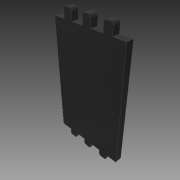
# Autodesk Inventor part: spool_stand_brace_middle_b
Saved by Autodesk Inventor 2014 (Build 180170000, 170)
## iProperties
Created: 2014-04-08
Part Number: spool_stand_brace_middle_b
Material: Plywood, Finish
Document SubType Name: Modeling
Designer: buben
Density: 0.552 g/cm^3
Appearance: Anodized - Dark Gray
Author: buben
Autodesk Inventor part; units mm, degrees
ref_plane "YZ Plane" through (0, 0, 0) normal (1, 0, 0) x (0, 1, 0)
ref_plane "XZ Plane" through (0, 0, 0) normal (0, 1, 0) x (-1, 0, 0)
ref_plane "XY Plane" through (0, 0, 0) normal (0, 0, 1) x (1, 0, 0)
sketch "Sketch1" plane through (0, 0, 0) normal (0, 1, 0) x (-1, 0, 0)
  line L0 (0, 0) -> (-68.411, 0)
  line L1 (-68.411, 0) -> (-68.411, -110)
  line L2 (-68.411, -110) -> (0, -110)
  line L3 (0, -110) -> (0, 0)
  dimension "d0" = 110
  dimension "d1" = 68.411
  constraints: 8 end point, 2 parallel, 1 horizontal, 1 perpendicular
  measures "d0" distance of L2.end L0.start
  measures "d1" distance of L0.start L0.end
extrude "Extrusion1" add sketch "Sketch1" along normal blind 6.5
sketch "Sketch2" plane through (0, 6.5, 0) normal (0, 1, 0) x (1, 0, 0)
  line L0 (68.411, 0) -> (68.411, 110) projected
  line L1 (68.411, 110) -> (0, 110) projected
  line L2 (0, 110) -> (0, 0) projected
  line L3 (11.1027, 110) -> (19.1027, 110)
  line L4 (19.1027, 110) -> (19.1027, 114.5)
  line L5 (17.1027, 116.5) -> (13.1027, 116.5)
  line L6 (11.1027, 114.5) -> (11.1027, 110)
  line L7 (30.2055, 110) -> (38.2055, 110)
  line L8 (38.2055, 110) -> (38.2055, 114.5)
  line L9 (36.2055, 116.5) -> (32.2055, 116.5)
  line L10 (30.2055, 114.5) -> (30.2055, 110)
  line L11 (49.3082, 110) -> (57.3082, 110)
  line L12 (57.3082, 110) -> (57.3082, 114.5)
  line L13 (55.3082, 116.5) -> (51.3082, 116.5)
  line L14 (49.3082, 114.5) -> (49.3082, 110)
  arc A0 (13.1027, 116.5) -> (11.1027, 114.5) centre (13.1027, 114.5) ccw
  arc A1 (19.1027, 114.5) -> (17.1027, 116.5) centre (17.1027, 114.5) ccw
  arc A2 (32.2055, 116.5) -> (30.2055, 114.5) centre (32.2055, 114.5) ccw
  arc A3 (38.2055, 114.5) -> (36.2055, 116.5) centre (36.2055, 114.5) ccw
  arc A4 (51.3082, 116.5) -> (49.3082, 114.5) centre (51.3082, 114.5) ccw
  arc A5 (57.3082, 114.5) -> (55.3082, 116.5) centre (55.3082, 114.5) ccw
  line L15 (11.1027, 112.25) -> (0, 112.25) construction
  line L16 (19.1027, 112.25) -> (30.2055, 112.25) construction
  line L17 (38.2055, 112.25) -> (49.3082, 112.25) construction
  line L18 (57.3082, 112.25) -> (68.411, 112.25) construction
  line L19 (0, 55) -> (68.411, 55) construction
  line L20 (0, 0) -> (68.411, 0) projected
  line L21 (68.411, 0) -> (68.411, 110) projected
  line L22 (68.411, 110) -> (0, 110) projected
  line L23 (0, 110) -> (0, 0) projected
  line L24 (11.1027, 0) -> (19.1027, 0)
  line L25 (19.1027, 0) -> (19.1027, -7.5)
  line L26 (17.1027, -9.5) -> (13.1027, -9.5)
  line L27 (11.1027, -7.5) -> (11.1027, 0)
  line L28 (30.2055, 0) -> (38.2055, 0)
  line L29 (38.2055, 0) -> (38.2055, -7.5)
  line L30 (36.2055, -9.5) -> (32.2055, -9.5)
  line L31 (30.2055, -7.5) -> (30.2055, 0)
  line L32 (49.3082, 0) -> (57.3082, 0)
  line L33 (57.3082, 0) -> (57.3082, -7.5)
  line L34 (55.3082, -9.5) -> (51.3082, -9.5)
  line L35 (49.3082, -7.5) -> (49.3082, 0)
  arc A6 (11.1027, -7.5) -> (13.1027, -9.5) centre (13.1027, -7.5) ccw
  arc A7 (17.1027, -9.5) -> (19.1027, -7.5) centre (17.1027, -7.5) ccw
  arc A8 (30.2055, -7.5) -> (32.2055, -9.5) centre (32.2055, -7.5) ccw
  arc A9 (36.2055, -9.5) -> (38.2055, -7.5) centre (36.2055, -7.5) ccw
  arc A10 (49.3082, -7.5) -> (51.3082, -9.5) centre (51.3082, -7.5) ccw
  arc A11 (55.3082, -9.5) -> (57.3082, -7.5) centre (55.3082, -7.5) ccw
  dimension "d4" = 2
  dimension "d5" = 8
  dimension "d6" = 8
  dimension "d7" = 8
  dimension "d8" = 6.5
  dimension "d11" = 2
  dimension "d12" = 9.5
  constraints: 58 end point, 24 point on circle, 24 tangent, 14 collinear, 12 centre point, 12 parallel, 10 equal radius, 8 midpoint, 7 perpendicular, 6 horizontal, 6 point on line, 2 vertical alignment
  measures "d4" radius of A0
  measures "d5" distance between parallel lines of L4 L6
  measures "d6" distance between parallel lines of L8 L10
  measures "d7" distance between parallel lines of L12 L14
  measures "d8" distance between parallel lines of L1 L5
  measures "d11" radius of A6
  measures "d12" distance between parallel lines of L26 L20
extrude "Extrusion3" add sketch "Sketch2" against normal blind 6.5 contours L33 A11 L34 A10 L35 L20 | L1 L14 A4 L13 A5 L12 | L29 A9 L30 A8 L31 L20 | L1 L10 A2 L9 A3 L8 | L25 A7 L26 A6 L27 L20 | L1 L6 A0 L5 A1 L4
equation "\"d6\" = d5"
equation "\"d7\" = d6"
body "Solid1"
